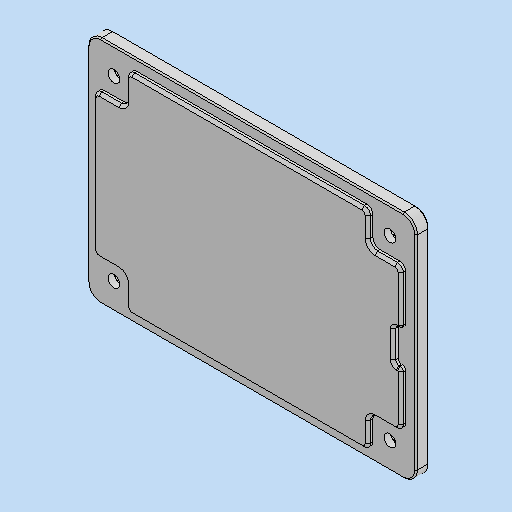
# Autodesk Inventor part: pump-box-lid
Saved by Autodesk Inventor 2025 (Build 290162000, 162)
## iProperties
Created: 2024-07-07
Part Number: pump-box-lid
Material: Generic
Document SubType Name: Modeling
Designer: queezz
Density: 1 g/cm^3
Appearance: Default
Author: queezz
Autodesk Inventor part; units mm, degrees
note: some values were not read from the file. Chosen so that the rebuilt part matches the saved one: direction of "Emboss1".
ref_plane "YZ Plane" through (0, 0, 0) normal (1, 0, 0) x (0, 1, 0)
ref_plane "XZ Plane" through (0, 0, 0) normal (0, 1, 0) x (-1, 0, 0)
ref_plane "XY Plane" through (0, 0, 0) normal (0, 0, 1) x (1, 0, 0)
sketch "Sketch1" plane through (0, 0, 0) normal (0, 0, 1) x (1, 0, 0)
  line L0 (-50, 35) -> (50, 35)
  line L1 (50, 35) -> (50, -35)
  line L2 (50, -35) -> (-50, -35)
  line L3 (-50, -35) -> (-50, 35)
  point P0 (0, 0)
  point P1 (50, 0)
  point P2 (0, 35)
  dimension "d0" = 100
  dimension "d1" = 70
  constraints: 8 end point, 2 midpoint, 2 parallel, 1 horizontal, 1 horizontal alignment, 1 perpendicular, 1 vertical alignment
  measures "d0" distance of L0.start L0.end
  measures "d1" distance of L0.end L1.end
extrude "Extrusion1" add sketch "Sketch1" along normal blind 4
fillet "Fillet1" radius 4 4 edges at (50, 35, 2) (50, -35, 2) (-50, 35, 2) (-50, -35, 2)
sketch "Sketch2" plane through (0, 0, 4) normal (0, 0, 1) x (1, 0, 0)
  line L0 (-42, 27) -> (42, 27) construction
  line L1 (42, 27) -> (42, -27) construction
  line L2 (42, -27) -> (-42, -27) construction
  line L3 (-42, -27) -> (-42, 27) construction
  line L4 (46, 35) -> (-46, 35) projected
  line L5 (-50, 31) -> (-50, -31) projected
  point P0 (0, 0)
  point P1 (42, 0)
  point P2 (0, 27)
  dimension "d48" = 8
  dimension "d49" = 8
  constraints: 8 end point, 4 coincident, 2 midpoint, 2 parallel, 1 horizontal, 1 horizontal alignment, 1 perpendicular, 1 vertical alignment
  measures "d48" distance between parallel lines of L4 L0
  measures "d49" distance between parallel lines of L5 L3
hole "Hole1" at (-42, 27, 4) at (42, 27, 4) at (42, -27, 4) at (-42, -27, 4) direction (0, 0, -1) diameter 3.6 depth 5 tip angle 118
sketch "Sketch3" plane through (0, 0, 4) normal (0, 0, 1) x (1, 0, 0)
  arc A0 (37, 24) -> (39, 22) centre (39, 24) ccw
  line L0 (37, 24) -> (37, 30)
  arc A1 (37, 30) -> (35, 32) centre (35, 30) ccw
  line L1 (35, 32) -> (-35, 32)
  arc A2 (-35, 32) -> (-37, 30) centre (-35, 30) ccw
  line L2 (-37, 30) -> (-37, 24)
  arc A3 (-39, 22) -> (-37, 24) centre (-39, 24) ccw
  line L3 (-39, 22) -> (-45, 22)
  arc A4 (-45, 22) -> (-47, 20) centre (-45, 20) ccw
  line L4 (-47, 20) -> (-47, -20)
  arc A5 (-47, -20) -> (-45, -22) centre (-45, -20) ccw
  line L5 (-45, -22) -> (-39, -22)
  arc A6 (-37, -24) -> (-39, -22) centre (-39, -24) ccw
  line L6 (-37, -24) -> (-37, -30)
  arc A7 (-37, -30) -> (-35, -32) centre (-35, -30) ccw
  line L7 (-35, -32) -> (35, -32)
  arc A8 (35, -32) -> (37, -30) centre (35, -30) ccw
  line L8 (37, -30) -> (37, -24)
  arc A9 (39, -22) -> (37, -24) centre (39, -24) ccw
  line L9 (39, -22) -> (45, -22)
  line L10 (45, 22) -> (39, 22)
  arc A10 (56, -27) -> (57, -26) centre (56, -26) ccw projected
  line L11 (57, -26) -> (56, -26) projected
  line L12 (56, -26) -> (56, -27) projected
  line L13 (50, -31) -> (50, 31) construction
  line L14 (-50, 31) -> (-50, -31) projected
  line L15 (0, -32) -> (0, 32) construction
  line L16 (47, 20) -> (47, -20)
  arc A11 (47, 20) -> (45, 22) centre (45, 20) ccw
  arc A12 (45, -22) -> (47, -20) centre (45, -20) ccw
  line L17 (46, 35) -> (-46, 35) projected
  point P0 (0, 0)
  point P1 (47, -22)
  point P2 (47, 22)
  point P3 (-37, 27)
  point P4 (-37, -27)
  point P5 (37, 27)
  point P6 (37, -27)
  point P7 (-47, 0)
  point P8 (0, 0)
  point P9 (60, 0)
  point P10 (47, 0)
  point P11 (42, -22)
  point P12 (-42, -22)
  dimension "d15" = 3
  dimension "d20" = 13
  dimension "d21" = 13
  dimension "d22" = 2
  dimension "d41" = 3
  dimension "d42" = 2
  dimension "d45" = 13
  dimension "d50" = 3
  constraints: 26 end point, 24 point on circle, 24 tangent, 12 centre point, 11 midpoint, 10 equal radius, 5 horizontal, 5 horizontal alignment, 5 vertical, 4 point on line, 2 vertical alignment
  measures "d15" distance between parallel lines of L14 L4
  measures "d20" distance between parallel lines of L13 L0
  measures "d21" distance from line of L14 point (-37, 27)
  measures "d22" radius of A3
  measures "d41" distance between parallel lines of L13 L16
  measures "d42" radius of A11
  measures "d45" distance between parallel lines of L10 L17
  measures "d50" distance between parallel lines of L17 L1
extrude "Extrusion2" add sketch "Sketch3" along normal blind 1.5 contours A0 L10 A11 L16 A12 L9 A9 L8 A8 L7 A7 L6 A6 L5 A5 L4 A4 L3 A3 L2 A2 L1 A1 L0
chamfer "Chamfer1" distance 0.4 angle 45 16 edges at (0, -35, 0) (48.8284, -33.8284, 0) (50, 0, 0) (48.8284, 33.8284, 0) (0, 35, 0) (-48.8284, 33.8284, 0) (-50, 0, 0) (-48.8284, -33.8284, 0) (0, -35, 4) (48.8284, -33.8284, 4) (50, 0, 4) (-48.8284, -33.8284, 4) (-50, 0, 4) (-48.8284, 33.8284, 4) (0, 35, 4) (48.8284, 33.8284, 4)
sketch "Sketch4" plane through (0, 0, 0) normal (0, 0, -1) x (-1, 0, 0)
  circle A0 centre (-42, 27) radius 1.8
  circle A1 centre (-42, -27) radius 1.8
  circle A2 centre (42, 27) radius 1.8
  circle A3 centre (42, -27) radius 1.8
  line L0 (-46, 35) -> (46, 35) projected
  line L1 (-50, -31) -> (-50, 31) projected
  line L2 (-42, 27) -> (42, 27) construction
  line L3 (42, 27) -> (42, -27) construction
  line L4 (42, -27) -> (-42, -27) construction
  line L5 (-42, -27) -> (-42, 27) construction
  point P0 (0, 0)
  point P1 (-42, 0)
  point P2 (0, -27)
  dimension "d46" = 8
  dimension "d47" = 8
  constraints: 8 end point, 6 coincident, 4 centre point, 2 midpoint, 2 parallel, 1 horizontal, 1 horizontal alignment, 1 perpendicular, 1 vertical alignment
  measures "d46" distance from line of L0 L2.start
  measures "d47" distance from line of L1 L2.start
hole "Hole2" at (42, 27, 0) at (42, -27, 0) at (-42, 27, 0) at (-42, -27, 0) direction (0, 0, 1) diameter 6.4 depth 2
sketch "Sketch5" plane through (-42, 27, 2) normal (0, 0, -1) x (-1, 0, 0)
  circle A0 centre (0, 0) radius 3.2 projected
  circle A1 centre (0, 0) radius 1.8 projected
  line L0 (2.6458, 1.8) -> (-2.6458, 1.8)
  line L1 (-2.6458, -1.8) -> (2.6458, -1.8)
  point P0 (-42, -27)
  point P1 (2.2875, -1.7)
  point P2 (-2.2875, 1.7)
  constraints: 4 end point, 4 point on circle, 2 tangent, 1 horizontal, 1 parallel
extrude "Extrusion3" add sketch "Sketch5" along normal blind 0.6 contours L0 A0 | A0 L1
sketch "Sketch6" plane through (-39.3542, 25.2, 2) normal (0, 0, -1) x (-1, 0, 0)
  arc A0 (0, 0) -> (5.2915, 0) centre (2.6458, 1.8) ccw projected
  line L0 (0.8458, -0.8458) -> (0.8458, 4.4458)
  circle A1 centre (2.6458, 1.8) radius 3.2 projected
  line L1 (4.4458, 4.4458) -> (4.4458, -0.8458)
  arc A2 (2.6458, 3.6) -> (2.6458, 0) centre (2.6458, 1.8) ccw projected
  arc A3 (2.6458, 0) -> (2.6458, 3.6) centre (2.6458, 1.8) ccw projected
  point P0 (-39.3542, -25.2)
  point P1 (4.2, -0.6)
  constraints: 4 end point, 4 point on circle, 2 tangent, 2 vertical
extrude "Extrusion5" add sketch "Sketch6" along normal blind 0.3 contours A1 L0 A0 | L1 A1 A0
mirror "Mirror1" about plane through (0, 0, 0) normal (1, 0, 0) of "Extrusion3", "Extrusion5"
mirror "Mirror2" about plane through (0, 0, 0) normal (0, 1, 0) of "Extrusion3", "Mirror1", "Extrusion5"
thicken "Thicken2" operation cut thickness 0.2 both sides no extend neighbours no toward (0, 1, 0) faces at (41, -22, 4.5) (46.1266, -21.6525, 5) (47, -6.6667, 4.5) (37.1383, -23.2693, 5) (37, -28, 4.5) (36.1266, -31.6525, 5) (-11.6667, -32, 4.5) (-36, -31.7321, 5) (-37, -26, 4.5) (-38.2693, -22.1383, 5) (-43, -22, 4.5) (-46.3603, -21.4661, 5) (-47, 6.6667, 4.5) (-46.4661, 21.3603, 5) (-41, 22, 4.5) (-37.6397, 22.5339, 5) (-37, 28, 4.5) (-36.7321, 31, 5) (11.6667, 32, 4.5) (36.1266, 31.6525, 5) (37, 26, 4.5) (37.0889, 23.4105, 5) (43, 22, 4.5) (46.6525, 21.1266, 5)
sketch "Sketch7" plane through (0, 0, 0) normal (0, 0, -1) x (-1, 0, 0)
  line L0 (30.2673, -23.5692) -> (30.2673, -3.5265) construction
  line L1 (30.2673, -3.5265) -> (37.3154, -3.5265) construction
  line L2 (37.3154, -3.5265) -> (37.3154, -23.5692) construction
  line L3 (37.3154, -23.5692) -> (30.2673, -23.5692) construction
  line L4 (-45.4551, 18.7248) -> (-45.4551, 8.6107) construction
  line L5 (-45.4551, 8.6107) -> (-38.3383, 8.6107) construction
  line L6 (-38.3383, 8.6107) -> (-38.3383, 18.7248) construction
  line L7 (-38.3383, 18.7248) -> (-45.4551, 18.7248) construction
  line L8 (-38.7348, -17.4978) -> (-45.0587, -17.4978) construction
  line L9 (-45.0587, -17.4978) -> (-45.0587, -9.0587) construction
  line L10 (-45.0587, -9.0587) -> (-38.7348, -9.0587) construction
  line L11 (-38.7348, -9.0587) -> (-38.7348, -17.4978) construction
  line L12 (29.1356, 3.2412) -> (29.1356, 23.2839) construction
  line L13 (29.1356, 23.2839) -> (36.1837, 23.2839) construction
  line L14 (36.1837, 23.2839) -> (36.1837, 3.2412) construction
  line L15 (36.1837, 3.2412) -> (29.1356, 3.2412) construction
  line L16 (30.8755, -18.0927) -> (35.0131, -18.0927)
  line L17 (35.0131, -18.0927) -> (35.0131, -19.4338)
  line L18 (35.0131, -19.4338) -> (34.3398, -19.4338)
  spline S0 degree 2 poles (34.3398, -19.4338) (34.7687, -19.727) (35.1706, -20.4438) (35.1706, -20.927) knots 0 0 0 1 2 2 2
  spline S1 degree 2 poles (35.1706, -20.927) (35.1706, -21.7578) (34.5624, -22.2519) knots 0 0 0 1 1 1
  spline S2 degree 2 poles (34.5624, -22.2519) (34.2638, -22.4908) (33.4547, -22.746) (32.9443, -22.746) knots 0 0 0 1 2 2 2
  spline S3 degree 2 poles (32.9443, -22.746) (31.9289, -22.746) (30.7398, -21.7035) (30.7398, -20.8293) knots 0 0 0 1 2 2 2
  spline S4 degree 2 poles (30.7398, -20.8293) (30.7398, -20.3623) (30.9407, -20.0257) knots 0 0 0 1 1 1
  spline S5 degree 2 poles (30.9407, -20.0257) (31.1362, -19.689) (31.5543, -19.4447) knots 0 0 0 1 1 1
  line L19 (31.5543, -19.4447) -> (30.8755, -19.4447)
  line L20 (30.8755, -19.4447) -> (30.8755, -18.0927)
  spline S6 degree 2 poles (32.9389, -19.3795) (32.4448, -19.3795) (32.1787, -19.6347) knots 0 0 0 1 1 1
  spline S7 degree 2 poles (32.1787, -19.6347) (31.8909, -19.9008) (31.8909, -20.3406) knots 0 0 0 1 1 1
  spline S8 degree 2 poles (31.8909, -20.3406) (31.8909, -20.7859) (32.1678, -21.0411) knots 0 0 0 1 1 1
  spline S9 degree 2 poles (32.1678, -21.0411) (32.4556, -21.3017) (32.9389, -21.3017) knots 0 0 0 1 1 1
  spline S10 degree 2 poles (32.9389, -21.3017) (33.4221, -21.3017) (33.7045, -21.0411) knots 0 0 0 1 1 1
  spline S11 degree 2 poles (33.7045, -21.0411) (33.976, -20.7913) (33.976, -20.3406) knots 0 0 0 1 1 1
  spline S12 degree 2 poles (33.976, -20.3406) (33.976, -19.9008) (33.4276, -19.3795) (32.9389, -19.3795) knots 0 0 0 1 2 2 2
  line L21 (35.0131, -11.5171) -> (32.7543, -11.5171)
  spline S13 degree 2 poles (32.7543, -11.5171) (32.2221, -11.5171) (32.0158, -11.642) knots 0 0 0 1 1 1
  spline S14 degree 2 poles (32.0158, -11.642) (31.8095, -11.7777) (31.8095, -12.1035) knots 0 0 0 1 1 1
  spline S15 degree 2 poles (31.8095, -12.1035) (31.8095, -12.5216) (32.0918, -12.6736) knots 0 0 0 1 1 1
  spline S16 degree 2 poles (32.0918, -12.6736) (32.3687, -12.8365) (33.2592, -12.8365) knots 0 0 0 1 1 1
  line L22 (33.2592, -12.8365) -> (35.0131, -12.8365)
  line L23 (35.0131, -12.8365) -> (35.0131, -14.2429)
  line L24 (35.0131, -14.2429) -> (32.7543, -14.2429)
  spline S17 degree 2 poles (32.7543, -14.2429) (32.2004, -14.2429) (32.0104, -14.3786) knots 0 0 0 1 1 1
  spline S18 degree 2 poles (32.0104, -14.3786) (31.8095, -14.5035) (31.8095, -14.8347) knots 0 0 0 1 1 1
  spline S19 degree 2 poles (31.8095, -14.8347) (31.8095, -15.2474) (32.081, -15.4157) knots 0 0 0 1 1 1
  spline S20 degree 2 poles (32.081, -15.4157) (32.3633, -15.5732) (33.2592, -15.5732) knots 0 0 0 1 1 1
  line L25 (33.2592, -15.5732) -> (35.0131, -15.5732)
  line L26 (35.0131, -15.5732) -> (35.0131, -16.9904)
  line L27 (35.0131, -16.9904) -> (30.8755, -16.9904)
  line L28 (30.8755, -16.9904) -> (30.8755, -15.5569)
  line L29 (30.8755, -15.5569) -> (31.5923, -15.5569)
  spline S21 degree 2 poles (31.5923, -15.5569) (31.1579, -15.2963) (30.9516, -14.9596) knots 0 0 0 1 1 1
  spline S22 degree 2 poles (30.9516, -14.9596) (30.7398, -14.6284) (30.7398, -14.1614) knots 0 0 0 1 1 1
  spline S23 degree 2 poles (30.7398, -14.1614) (30.7398, -13.6565) (30.9353, -13.3307) knots 0 0 0 1 1 1
  spline S24 degree 2 poles (30.9353, -13.3307) (31.1307, -13.0212) (31.5217, -12.88) knots 0 0 0 1 1 1
  spline S25 degree 2 poles (31.5217, -12.88) (31.1144, -12.6248) (30.9353, -12.2827) knots 0 0 0 1 1 1
  spline S26 degree 2 poles (30.9353, -12.2827) (30.7398, -11.9406) (30.7398, -11.4628) knots 0 0 0 1 1 1
  spline S27 degree 2 poles (30.7398, -11.4628) (30.7398, -11.0881) (30.8647, -10.8112) knots 0 0 0 1 1 1
  spline S28 degree 2 poles (30.8647, -10.8112) (31.0004, -10.5234) (31.2393, -10.3388) knots 0 0 0 1 1 1
  spline S29 degree 2 poles (31.2393, -10.3388) (31.4348, -10.1813) (31.6954, -10.1162) knots 0 0 0 1 1 1
  spline S30 degree 2 poles (31.6954, -10.1162) (31.9398, -10.0565) (32.5534, -10.0565) knots 0 0 0 1 1 1
  line L30 (32.5534, -10.0565) -> (32.6402, -10.0565)
  line L31 (32.6402, -10.0565) -> (35.0131, -10.0565)
  line L32 (35.0131, -10.0565) -> (35.0131, -11.5171)
  line L33 (36.843, -9.0193) -> (30.881, -9.0193)
  line L34 (30.881, -9.0193) -> (30.881, -7.6782)
  line L35 (30.881, -7.6782) -> (31.5706, -7.6782)
  spline S31 degree 2 poles (31.5706, -7.6782) (31.1742, -7.4121) (30.9516, -7.0537) knots 0 0 0 1 1 1
  spline S32 degree 2 poles (30.9516, -7.0537) (30.7506, -6.7117) (30.7506, -6.2773) knots 0 0 0 1 1 1
  spline S33 degree 2 poles (30.7506, -6.2773) (30.7506, -5.8374) (31.0439, -5.1424) (31.3371, -4.8818) knots 0 0 0 1 2 2 2
  spline S34 degree 2 poles (31.3371, -4.8818) (31.9235, -4.3714) (32.9552, -4.3714) knots 0 0 0 1 1 1
  spline S35 degree 2 poles (32.9552, -4.3714) (33.9434, -4.3714) (34.557, -4.8818) knots 0 0 0 1 1 1
  spline S36 degree 2 poles (34.557, -4.8818) (34.8665, -5.1479) (35.1706, -5.8049) (35.1706, -6.2284) knots 0 0 0 1 2 2 2
  spline S37 degree 2 poles (35.1706, -6.2284) (35.1706, -6.7551) (34.9751, -7.0863) knots 0 0 0 1 1 1
  spline S38 degree 2 poles (34.9751, -7.0863) (34.7905, -7.4012) (34.3398, -7.6727) knots 0 0 0 1 1 1
  spline S39 degree 2 poles (34.3398, -7.6727) (34.4375, -7.651) (34.6384, -7.6347) knots 0 0 0 1 1 1
  spline S40 degree 2 poles (34.6384, -7.6347) (34.7579, -7.6293) (35.0782, -7.6293) knots 0 0 0 1 1 1
  line L36 (35.0782, -7.6293) -> (36.843, -7.6293)
  line L37 (36.843, -7.6293) -> (36.843, -9.0193)
  spline S41 degree 2 poles (32.9552, -7.727) (33.4384, -7.727) (33.7208, -7.4718) knots 0 0 0 1 1 1
  spline S42 degree 2 poles (33.7208, -7.4718) (33.9923, -7.2329) (33.9923, -6.7877) knots 0 0 0 1 1 1
  spline S43 degree 2 poles (33.9923, -6.7877) (33.9923, -6.3424) (33.7208, -6.0927) knots 0 0 0 1 1 1
  spline S44 degree 2 poles (33.7208, -6.0927) (33.433, -5.8429) (32.9552, -5.8429) knots 0 0 0 1 1 1
  spline S45 degree 2 poles (32.9552, -5.8429) (32.4719, -5.8429) (32.195, -6.0927) knots 0 0 0 1 1 1
  spline S46 degree 2 poles (32.195, -6.0927) (31.9181, -6.3424) (31.9181, -6.7877) knots 0 0 0 1 1 1
  spline S47 degree 2 poles (31.9181, -6.7877) (31.9181, -7.2275) (32.195, -7.4718) knots 0 0 0 1 1 1
  spline S48 degree 2 poles (32.195, -7.4718) (32.4665, -7.727) (32.9552, -7.727) knots 0 0 0 1 1 1
  line L38 (-38.8967, -14.1063) -> (-44.8967, -14.1063)
  line L39 (-44.8967, -14.1063) -> (-44.8967, -12.4557)
  line L40 (-44.8967, -12.4557) -> (-38.8967, -12.4557)
  line L41 (-38.8967, -12.4557) -> (-38.8967, -14.1063)
  line L42 (-44.8967, 14.4497) -> (-38.8967, 16.9637)
  line L43 (-38.8967, 16.9637) -> (-38.8967, 15.2261)
  line L44 (-38.8967, 15.2261) -> (-42.2524, 14.0261)
  spline S49 degree 2 poles (-42.2524, 14.0261) (-42.2525, 14.0261) (-42.3664, 13.999) (-42.5022, 13.961) knots 0 0 0 1 2 2 2
  spline S50 degree 2 poles (-42.5022, 13.961) (-42.7139, 13.9121) (-43.056, 13.8252) knots 0 0 0 1 1 1
  spline S51 degree 2 poles (-43.056, 13.8252) (-42.8117, 13.7709) (-42.5619, 13.7004) knots 0 0 0 1 1 1
  spline S52 degree 2 poles (-42.5619, 13.7004) (-42.323, 13.6461) (-42.2524, 13.6189) knots 0 0 0 1 1 1
  line L45 (-42.2524, 13.6189) -> (-38.8967, 12.4243)
  line L46 (-38.8967, 12.4243) -> (-38.8967, 10.6868)
  line L47 (-38.8967, 10.6868) -> (-44.8967, 13.2008)
  line L48 (-44.8967, 13.2008) -> (-44.8967, 14.4497)
  line L49 (36.7511, 1.2137) -> (30.7891, 1.2137)
  line L50 (30.7891, 1.2137) -> (30.7891, 2.5549)
  line L51 (30.7891, 2.5549) -> (31.4787, 2.5549)
  spline S53 degree 2 poles (31.4787, 2.5549) (31.0823, 2.8209) (30.8597, 3.1793) knots 0 0 0 1 1 1
  spline S54 degree 2 poles (30.8597, 3.1793) (30.6588, 3.5214) (30.6588, 3.9558) knots 0 0 0 1 1 1
  spline S55 degree 2 poles (30.6588, 3.9558) (30.6588, 4.3956) (30.952, 5.0906) (31.2452, 5.3512) knots 0 0 0 1 2 2 2
  spline S56 degree 2 poles (31.2452, 5.3512) (31.8316, 5.8616) (32.8633, 5.8616) knots 0 0 0 1 1 1
  spline S57 degree 2 poles (32.8633, 5.8616) (33.8515, 5.8616) (34.4651, 5.3512) knots 0 0 0 1 1 1
  spline S58 degree 2 poles (34.4651, 5.3512) (34.7746, 5.0852) (35.0787, 4.4282) (35.0787, 4.0046) knots 0 0 0 1 2 2 2
  spline S59 degree 2 poles (35.0787, 4.0046) (35.0787, 3.4779) (34.8832, 3.1467) knots 0 0 0 1 1 1
  spline S60 degree 2 poles (34.8832, 3.1467) (34.6986, 2.8318) (34.2479, 2.5603) knots 0 0 0 1 1 1
  spline S61 degree 2 poles (34.2479, 2.5603) (34.3457, 2.582) (34.5466, 2.5983) knots 0 0 0 1 1 1
  spline S62 degree 2 poles (34.5466, 2.5983) (34.666, 2.6037) (34.9864, 2.6037) knots 0 0 0 1 1 1
  line L52 (34.9864, 2.6037) -> (36.7511, 2.6037)
  line L53 (36.7511, 2.6037) -> (36.7511, 1.2137)
  spline S63 degree 2 poles (32.8633, 2.506) (33.3466, 2.506) (33.6289, 2.7612) knots 0 0 0 1 1 1
  spline S64 degree 2 poles (33.6289, 2.7612) (33.9004, 3.0001) (33.9004, 3.4454) knots 0 0 0 1 1 1
  spline S65 degree 2 poles (33.9004, 3.4454) (33.9004, 3.8906) (33.6289, 4.1404) knots 0 0 0 1 1 1
  spline S66 degree 2 poles (33.6289, 4.1404) (33.3411, 4.3901) (32.8633, 4.3901) knots 0 0 0 1 1 1
  spline S67 degree 2 poles (32.8633, 4.3901) (32.3801, 4.3901) (32.1031, 4.1404) knots 0 0 0 1 1 1
  spline S68 degree 2 poles (32.1031, 4.1404) (31.8262, 3.8906) (31.8262, 3.4454) knots 0 0 0 1 1 1
  spline S69 degree 2 poles (31.8262, 3.4454) (31.8262, 3.0055) (32.1031, 2.7612) knots 0 0 0 1 1 1
  spline S70 degree 2 poles (32.1031, 2.7612) (32.3746, 2.506) (32.8633, 2.506) knots 0 0 0 1 1 1
  line L54 (34.9212, 6.7521) -> (30.7837, 6.7521)
  line L55 (30.7837, 6.7521) -> (30.7837, 8.1313)
  line L56 (30.7837, 8.1313) -> (31.761, 8.1313)
  spline S71 degree 2 poles (31.761, 8.1313) (31.2235, 8.3485) (30.9574, 8.7123) knots 0 0 0 1 1 1
  spline S72 degree 2 poles (30.9574, 8.7123) (30.6914, 9.0816) (30.6914, 9.6082) knots 0 0 0 1 1 1
  spline S73 degree 2 poles (30.6914, 9.6082) (30.6914, 9.7277) (30.6968, 9.7874) knots 0 0 0 1 1 1
  spline S74 degree 2 poles (30.6968, 9.7874) (30.7022, 9.8309) (30.7022, 9.9015) (30.7131, 9.9612) knots 0 0 0 1 2 2 2
  line L57 (30.7131, 9.9612) -> (32.0488, 9.82)
  spline S75 degree 2 poles (32.0488, 9.82) (32, 9.668) (31.9782, 9.5594) knots 0 0 0 1 1 1
  spline S76 degree 2 poles (31.9782, 9.5594) (31.962, 9.3965) (31.962, 9.3205) knots 0 0 0 1 1 1
  spline S77 degree 2 poles (31.962, 9.3205) (31.962, 8.7829) (32.2877, 8.4951) knots 0 0 0 1 1 1
  spline S78 degree 2 poles (32.2877, 8.4951) (32.6135, 8.2073) (33.2108, 8.2073) knots 0 0 0 1 1 1
  line L58 (33.2108, 8.2073) -> (34.9212, 8.2073)
  line L59 (34.9212, 8.2073) -> (34.9212, 6.7521)
  spline S79 degree 2 poles (32.8633, 14.8915) (33.314, 14.8915) (33.7104, 14.7178) knots 0 0 0 1 1 1
  spline S80 degree 2 poles (33.7104, 14.7178) (34.1285, 14.5331) (34.4325, 14.2128) knots 0 0 0 1 1 1
  spline S81 degree 2 poles (34.4325, 14.2128) (34.7692, 13.849) (34.9212, 13.4635) knots 0 0 0 1 1 1
  spline S82 degree 2 poles (34.9212, 13.4635) (35.0787, 13.0616) (35.0787, 12.573) knots 0 0 0 1 1 1
  spline S83 degree 2 poles (35.0787, 12.573) (35.0787, 12.0843) (34.9212, 11.6825) knots 0 0 0 1 1 1
  spline S84 degree 2 poles (34.9212, 11.6825) (34.7583, 11.2806) (34.1068, 10.5911) (33.7104, 10.439) knots 0 0 0 1 2 2 2
  spline S85 degree 2 poles (33.7104, 10.439) (33.3303, 10.2653) (32.8633, 10.2653) knots 0 0 0 1 1 1
  spline S86 degree 2 poles (32.8633, 10.2653) (32.4072, 10.2653) (32.0054, 10.439) knots 0 0 0 1 1 1
  spline S87 degree 2 poles (32.0054, 10.439) (31.5982, 10.6073) (31.2832, 10.9386) knots 0 0 0 1 1 1
  spline S88 degree 2 poles (31.2832, 10.9386) (30.9737, 11.2589) (30.8054, 11.6825) knots 0 0 0 1 1 1
  spline S89 degree 2 poles (30.8054, 11.6825) (30.6479, 12.0843) (30.6479, 12.573) knots 0 0 0 1 1 1
  spline S90 degree 2 poles (30.6479, 12.573) (30.6479, 13.0562) (30.8054, 13.4635) knots 0 0 0 1 1 1
  spline S91 degree 2 poles (30.8054, 13.4635) (30.9737, 13.887) (31.2832, 14.2073) knots 0 0 0 1 1 1
  spline S92 degree 2 poles (31.2832, 14.2073) (31.5927, 14.5494) (32.0054, 14.7123) knots 0 0 0 1 1 1
  spline S93 degree 2 poles (32.0054, 14.7123) (32.4072, 14.8915) (32.8633, 14.8915) knots 0 0 0 1 1 1
  spline S94 degree 2 poles (32.8579, 13.4363) (32.3963, 13.4363) (32.1303, 13.2028) knots 0 0 0 1 1 1
  spline S95 degree 2 poles (32.1303, 13.2028) (31.8642, 12.9639) (31.8642, 12.573) knots 0 0 0 1 1 1
  spline S96 degree 2 poles (31.8642, 12.573) (31.8642, 12.1711) (32.1303, 11.9431) knots 0 0 0 1 1 1
  spline S97 degree 2 poles (32.1303, 11.9431) (32.3909, 11.7096) (32.8579, 11.7096) knots 0 0 0 1 1 1
  spline S98 degree 2 poles (32.8579, 11.7096) (33.3194, 11.7096) (33.5801, 11.9322) knots 0 0 0 1 1 1
  spline S99 degree 2 poles (33.5801, 11.9322) (33.8515, 12.182) (33.8515, 12.573) knots 0 0 0 1 1 1
  spline S100 degree 2 poles (33.8515, 12.573) (33.8515, 12.9639) (33.5801, 13.2137) knots 0 0 0 1 1 1
  spline S101 degree 2 poles (33.5801, 13.2137) (33.3086, 13.4363) (32.8579, 13.4363) knots 0 0 0 1 1 1
  line L60 (28.5683, 15.7386) -> (28.5683, 17.1286)
  line L61 (28.5683, 17.1286) -> (30.7348, 17.1286)
  spline S102 degree 2 poles (30.7348, 17.1286) (31.0497, 17.1286) (31.1692, 17.1232) knots 0 0 0 1 1 1
  spline S103 degree 2 poles (31.1692, 17.1232) (31.381, 17.1015) (31.4678, 17.0852) knots 0 0 0 1 1 1
  spline S104 degree 2 poles (31.4678, 17.0852) (31.0226, 17.3458) (30.8434, 17.6716) knots 0 0 0 1 1 1
  spline S105 degree 2 poles (30.8434, 17.6716) (30.6479, 17.9974) (30.6479, 18.5295) knots 0 0 0 1 1 1
  spline S106 degree 2 poles (30.6479, 18.5295) (30.6479, 19.3549) (31.2506, 19.8761) knots 0 0 0 1 1 1
  spline S107 degree 2 poles (31.2506, 19.8761) (31.8588, 20.3865) (32.8525, 20.3865) knots 0 0 0 1 1 1
  spline S108 degree 2 poles (32.8525, 20.3865) (33.8733, 20.3865) (34.4706, 19.8761) knots 0 0 0 1 1 1
  spline S109 degree 2 poles (34.4706, 19.8761) (35.0787, 19.3549) (35.0787, 18.4806) knots 0 0 0 1 1 1
  spline S110 degree 2 poles (35.0787, 18.4806) (35.0787, 18.0408) (34.8724, 17.7042) knots 0 0 0 1 1 1
  spline S111 degree 2 poles (34.8724, 17.7042) (34.6715, 17.3567) (34.2479, 17.0797) knots 0 0 0 1 1 1
  line L62 (34.2479, 17.0797) -> (34.9212, 17.0797)
  line L63 (34.9212, 17.0797) -> (34.9212, 15.7386)
  line L64 (34.9212, 15.7386) -> (28.5683, 15.7386)
  spline S112 degree 2 poles (32.8525, 17.0309) (33.352, 17.0309) (33.6181, 17.2861) knots 0 0 0 1 1 1
  spline S113 degree 2 poles (33.6181, 17.2861) (33.895, 17.525) (33.895, 17.9702) knots 0 0 0 1 1 1
  spline S114 degree 2 poles (33.895, 17.9702) (33.895, 18.4155) (33.3466, 18.915) (32.8525, 18.915) knots 0 0 0 1 2 2 2
  spline S115 degree 2 poles (32.8525, 18.915) (32.3692, 18.915) (32.0923, 18.6653) knots 0 0 0 1 1 1
  spline S116 degree 2 poles (32.0923, 18.6653) (31.8153, 18.4155) (31.8153, 17.9702) knots 0 0 0 1 1 1
  spline S117 degree 2 poles (31.8153, 17.9702) (31.8153, 17.5304) (32.0923, 17.2861) knots 0 0 0 1 1 1
  spline S118 degree 2 poles (32.0923, 17.2861) (32.3638, 17.0309) (32.8525, 17.0309) knots 0 0 0 1 1 1
  line L65 (33.1402, 25.5612) -> (33.1402, 22.4173)
  spline S119 degree 2 poles (33.1402, 22.4173) (33.6235, 22.4282) (33.8787, 22.6562) knots 0 0 0 1 1 1
  spline S120 degree 2 poles (33.8787, 22.6562) (34.1393, 22.8951) (34.1393, 23.3458) knots 0 0 0 1 1 1
  spline S121 degree 2 poles (34.1393, 23.3458) (34.1393, 23.6716) (34.0144, 23.9051) knots 0 0 0 1 1 1
  spline S122 degree 2 poles (34.0144, 23.9051) (33.8787, 24.144) (33.6452, 24.2526) knots 0 0 0 1 1 1
  line L66 (33.6452, 24.2526) -> (34.085, 25.3494)
  spline S123 degree 2 poles (34.085, 25.3494) (34.5574, 25.154) (34.8181, 24.6544) knots 0 0 0 1 1 1
  spline S124 degree 2 poles (34.8181, 24.6544) (35.0787, 24.1494) (35.0787, 23.4273) knots 0 0 0 1 1 1
  spline S125 degree 2 poles (35.0787, 23.4273) (35.0787, 22.3467) (34.4706, 21.6897) knots 0 0 0 1 1 1
  spline S126 degree 2 poles (34.4706, 21.6897) (33.8841, 21.0381) (32.8959, 21.0381) knots 0 0 0 1 1 1
  spline S127 degree 2 poles (32.8959, 21.0381) (31.9294, 21.0381) (31.2832, 21.6897) knots 0 0 0 1 1 1
  spline S128 degree 2 poles (31.2832, 21.6897) (30.6479, 22.3413) (30.6479, 23.3458) knots 0 0 0 1 1 1
  spline S129 degree 2 poles (30.6479, 23.3458) (30.6479, 24.3666) (31.2941, 24.9639) knots 0 0 0 1 1 1
  spline S130 degree 2 poles (31.2941, 24.9639) (31.6253, 25.268) (32.5049, 25.5612) (33.0696, 25.5612) knots 0 0 0 1 2 2 2
  line L67 (33.0696, 25.5612) -> (33.1402, 25.5612)
  spline S131 degree 2 poles (32.3203, 24.1223) (31.9728, 24.0843) (31.5384, 23.6282) (31.5384, 23.2969) knots 0 0 0 1 2 2 2
  spline S132 degree 2 poles (31.5384, 23.2969) (31.5384, 22.9494) (31.7339, 22.7322) knots 0 0 0 1 1 1
  spline S133 degree 2 poles (31.7339, 22.7322) (31.9511, 22.5042) (32.3203, 22.4499) knots 0 0 0 1 1 1
  line L68 (32.3203, 22.4499) -> (32.3203, 24.1223)
  point P0 (0, 0)
  point P1 (-41.8967, 8.6107)
  point P2 (-41.8967, -9.0587)
  constraints: 2 midpoint, 1 vertical alignment, 8 other
emboss "Emboss1" sketch "Sketch7" operation cut depth 0.6 direction (0, 0, 1)
sketch "Sketch8" plane through (0, 0, 5.5) normal (0, 0, 1) x (1, 0, 0)
  line L0 (46.8, -20) -> (46.8, 20) projected
  line L1 (46.8, 5.15) -> (44.5, 5.15)
  line L2 (44.5, 5.15) -> (44.5, -5.15)
  line L3 (44.5, -5.15) -> (46.8, -5.15)
  line L4 (46.8, -5.15) -> (46.8, 5.15)
  point P0 (0, 0)
  point P1 (46.8, 0)
  dimension "d56" = 10.3
  dimension "d57" = 2.3
  constraints: 8 end point, 2 midpoint, 2 parallel, 1 horizontal, 1 perpendicular, 1 point on line
  measures "d56" distance of L1.end L2.end
  measures "d57" distance of L2.end L3.end
extrude "Extrusion6" cut sketch "Sketch8" against normal up to surface (1.5 mm away)
fillet "Fillet2" radius 1 4 edges at (46.8, 5.15, 4.75) (44.5, 5.15, 4.75) (44.5, -5.15, 4.75) (46.8, -5.15, 4.75)
chamfer "Chamfer2" distance 0.8 angle 45 23 edges at (0, 31.8, 5.5) (-42, -21.8, 5.5) (46.2728, 21.2728, 5.5) (37.4444, 22.4444, 5.5) (-36.2728, 31.2728, 5.5) (-37.4444, 22.4444, 5.5) (-46.2728, 21.2728, 5.5) (-37.4444, -22.4444, 5.5) (-36.8, 27, 5.5) (46.2728, -21.2728, 5.5) (37.4444, -22.4444, 5.5) (36.2728, -31.2728, 5.5) (42, -21.8, 5.5) (-42, 21.8, 5.5) (-46.8, 0, 5.5) (36.2728, 31.2728, 5.5) (-46.2728, -21.2728, 5.5) (-36.2728, -31.2728, 5.5) (0, -31.8, 5.5) (36.8, -27, 5.5) (-36.8, -27, 5.5) (42, 21.8, 5.5) (36.8, 27, 5.5)
body "Solid1"
